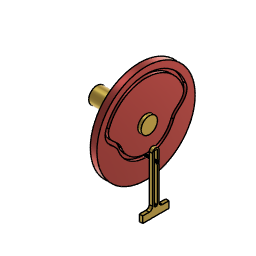
Groove Cam & Follower v1 (Autodesk Fusion 360 design; units mm, degrees)
Autodesk Fusion 360 part; units mm, degrees
sketch "Sketch1" plane through (0, 0, 0) normal (1, 0, 0) x (0, 1, 0) in component "Cam"
  circle A0 centre (0, 0) radius 150
  circle A1 centre (0, 0) radius 25
  line L0 (0, 0) -> (140.9539, 51.303) construction
  line L1 (0, 0) -> (150, 0) construction
  line L2 (0, 0) -> (140.9539, -51.303) construction
  line L3 (0, 0) -> (150, 0) construction
  line L4 (0, 0) -> (0, 44.9375) construction
  line L5 (0, 0) -> (-140.9539, 51.303) construction
  line L6 (0, 0) -> (-140.9539, -51.303) construction
  arc A2 (-84.5723, -30.7818) -> (84.5723, -30.7818) centre (0, 0) ccw
  arc A3 (-75.1754, -27.3616) -> (75.1754, -27.3616) centre (0, 0) ccw
  arc A4 (-79.8739, -29.0717) -> (79.8739, -29.0717) centre (0, 0) ccw construction
  arc A5 (112.7631, 41.0424) -> (-112.7631, 41.0424) centre (0, 0) ccw
  arc A6 (117.4616, 42.7525) -> (-117.4616, 42.7525) centre (0, 0) ccw construction
  arc A7 (122.16, 44.4626) -> (-122.16, 44.4626) centre (0, 0) ccw
  circle A8 centre (0, 0) radius 105 construction
  spline S0 degree 5 poles (79.8739, -29.0717) (80.4472, -27.4965) (81.7231, -24.4709) (84.0245, -20.3068) (87.8255, -15.4257) (93.5361, -10.0122) (99.8269, -4.7519) (106.2212, 0.8826) (112.1495, 7.2873) (116.9595, 14.6336) (119.9758, 22.9706) (120.4495, 30.4174) (119.4921, 36.4235) (118.2406, 40.6121) (117.4616, 42.7525) knots 0 0 0 0 0 0 0.1 0.2 0.3 0.4 0.5 0.6 0.7 0.8 0.9 1 1 1 1 1 1
  line L7 (76.7297, -37.7103) -> (83.0181, -20.4331)
  line L8 (121.1912, 32.5055) -> (113.732, 52.9996)
  spline S1 degree 3 poles (75.1754, -27.3616) (76.823, -22.8348) (79.1122, -18.7939) (81.8342, -15.2645) (86.0599, -9.7852) (91.2337, -5.5228) (96.2009, -1.2084) (100.1964, 2.262) (104.0844, 5.8134) (107.2713, 9.7654) (110.6099, 13.9054) (113.1413, 18.4168) (114.2898, 23.367) (115.4903, 28.5416) (115.2334, 34.2554) (112.7631, 41.0424) knots 0 0 0 0 0.154395 0.154395 0.154395 0.394087 0.394087 0.394087 0.586886 0.586886 0.586886 0.788862 0.788862 0.788862 1 1 1 1
  spline S2 degree 3 poles (84.5723, -30.7818) (86.6822, -24.985) (89.9, -20.6359) (94.2784, -16.3408) (97.8857, -12.8021) (102.2844, -9.3109) (106.7575, -5.2037) (111.1537, -1.1672) (115.5974, 3.4844) (119.026, 9.0954) (121.919, 13.8298) (124.0666, 19.2656) (124.7475, 25.2663) (125.3462, 30.5417) (124.7871, 36.2094) (122.9756, 42.0453) (122.7266, 42.8476) (122.4546, 43.6534) (122.16, 44.4626) knots 0 0 0 0 0.25 0.25 0.25 0.455973 0.455973 0.455973 0.6584 0.6584 0.6584 0.8292 0.8292 0.8292 0.979357 0.979357 0.979357 1 1 1 1
  spline S3 degree 3 poles (-75.1754, -27.3616) (-76.823, -22.8348) (-79.1122, -18.7939) (-81.8342, -15.2645) (-86.0599, -9.7852) (-91.2337, -5.5228) (-96.2009, -1.2084) (-100.1964, 2.262) (-104.0844, 5.8134) (-107.2713, 9.7654) (-110.6099, 13.9054) (-113.1413, 18.4168) (-114.2898, 23.367) (-115.4903, 28.5416) (-115.2334, 34.2554) (-112.7631, 41.0424) knots 0 0 0 0 0.154395 0.154395 0.154395 0.394087 0.394087 0.394087 0.586886 0.586886 0.586886 0.788862 0.788862 0.788862 1 1 1 1
  spline S4 degree 3 poles (-84.5723, -30.7818) (-86.6822, -24.985) (-89.9, -20.6359) (-94.2784, -16.3408) (-97.8857, -12.8021) (-102.2844, -9.3109) (-106.7575, -5.2037) (-111.1537, -1.1672) (-115.5974, 3.4844) (-119.026, 9.0954) (-121.919, 13.8298) (-124.0666, 19.2656) (-124.7475, 25.2663) (-125.3462, 30.5417) (-124.7871, 36.2094) (-122.9756, 42.0453) (-122.7266, 42.8476) (-122.4546, 43.6534) (-122.16, 44.4626) knots 0 0 0 0 0.25 0.25 0.25 0.455973 0.455973 0.455973 0.6584 0.6584 0.6584 0.8292 0.8292 0.8292 0.979357 0.979357 0.979357 1 1 1 1
  point P0 (105, 0)
  dimension "d1" = 300
  dimension "d4" = 160
  dimension "d5" = 180
  dimension "d6" = 50
  dimension "d8" = 170
  dimension "d9" = 20
  dimension "d10" = 20
  dimension "d11" = 150
  dimension "d12" = 210
  dimension "d13" = -5
  dimension "d14" = 5
  constraint coincident A0.centre A1.centre
  constraint concentric A1 A3
  constraint horizontal L1
  constraint horizontal L3
  constraint perpendicular L3 L4
  constraint symmetric A0.centre L4 A1.centre
  constraint symmetric L0.end L4 L5.end
  constraint symmetric L2.end L4 L6.end
  constraint coincident L6 A3.start
  constraint coincident L6 A2.start
  constraint coincident L5 A5.end
  constraint coincident L5 A6.end
  constraint coincident L5 A7.end
  constraint coincident L6 A4.start
  constraint coincident L0 A5.start
  constraint coincident L0 A6.start
  constraint coincident L0 A7.start
  constraint coincident L2 A2.end
  constraint coincident L2 A4.end
  constraint coincident L2 A3.end
  constraint concentric A1 A8
  constraint coincident A8 P0
  constraint coincident L1 P0
  constraint midpoint A4.end L7
  constraint tangent A4 L7
  constraint midpoint A6.start L8
  constraint tangent A6 L8
  constraint symmetric L4 A3.end A3.start
  constraint symmetric L4 A5.start A5.end
  constraint symmetric L4 S1 S3
  constraint symmetric L4 A2.end A2.start
  constraint symmetric L4 A7.start A7.end
  constraint symmetric L4 S2 S4
  measures "d1" diameter of A0
  measures "d4" diameter of A3
  measures "d5" diameter of A2
  measures "d6" diameter of A1
  measures "d8" diameter of A4
  measures "d9" angle of L0 L1
  measures "d10" angle of L2 L3
  measures "d11" distance of A0.centre L2.end
  measures "d12" diameter of A8
extrude "Extrude1" add sketch "Sketch1" along normal blind 20 makes body 1 at (0, -77.0806, 24.22) makes body 2 at (0, -121.0179, -46.6925) in component "Cam"
extrude "Extrude2" add sketch "Sketch1" along normal blind 10 contours A2 A7 S2 S4 bodies 1 2 in component "Cam"
cylinder "CylinderPrimitive1" add diameter 50 height -150 placed x (0, 0, -1) y (0, 1, 0) z (1, 0, 0) at (20, 0, 0) separate body makes body 3 in component "Axis"
move_face "OffsetFaces1" offset 10 1 faces at (20, -1.242, 6.7759) on bodies 3 in component "Axis"
ref_plane "WorkPlane1" through (50, 0, 20) normal (1, 0, 0) x (0, 1, 0) in component "Follower Base"
sketch "Sketch1 (2)" plane through (50, 0, 0) normal (1, 0, 0) x (0, 1, 0) in component "Follower Base"
  line L0 (10, -60) -> (10, -200)
  line L1 (-10, -200) -> (-10, -60)
  circle A0 centre (0, 0) radius 25
  line L2 (40, -210) -> (40, -230)
  line L3 (40, -230) -> (-40, -230)
  line L4 (-40, -230) -> (-40, -210)
  line L5 (4.8, -57.2) -> (4.8, -202.8)
  line L6 (2.8, -204.8) -> (-2.8, -204.8)
  line L7 (-4.8, -202.8) -> (-4.8, -57.2)
  line L8 (-2.8, -55.2) -> (2.8, -55.2)
  line L9 (-40, -210) -> (-20, -210)
  line L10 (20, -210) -> (40, -210)
  arc A1 (0, -50) -> (-10, -60) centre (0, -60) ccw
  arc A2 (10, -60) -> (0, -50) centre (0, -60) ccw
  arc A3 (-2.8, -55.2) -> (-4.8, -57.2) centre (-2.8, -57.2) ccw
  arc A4 (4.8, -57.2) -> (2.8, -55.2) centre (2.8, -57.2) ccw
  arc A5 (-4.8, -202.8) -> (-2.8, -204.8) centre (-2.8, -202.8) ccw
  arc A6 (2.8, -204.8) -> (4.8, -202.8) centre (2.8, -202.8) ccw
  arc A7 (-20, -210) -> (-10, -200) centre (-20, -200) ccw
  arc A8 (10, -200) -> (20, -210) centre (20, -200) ccw
  point P0 (-10, -50)
  point P1 (10, -50)
  point P2 (-10, -210)
  dimension "d23" = 20
  dimension "d24" = 160
  dimension "d25" = 10
  dimension "d27" = 80
  dimension "d28" = 20
  dimension "d29" = 30
  dimension "d31" = 10
  dimension "d32" = 2
  dimension "d33" = 2
  dimension "d34" = 10
  constraint vertical L0
  constraint vertical L1
  constraint horizontal L9
  constraint vertical L2
  constraint horizontal L3
  constraint vertical L4
  constraint collinear L9 L10
  constraint coincident P0 L1
  constraint tangent L1 A1
  constraint coincident P1 L0
  constraint tangent L0 A2
  constraint equal A1 A2
  constraint coincident A1.start A2.end
  constraint tangent L7 A3
  constraint tangent L8 A3
  constraint tangent L5 A4
  constraint tangent L8 A4
  constraint equal A3 A4
  constraint tangent L6 A5
  constraint tangent L7 A5
  constraint tangent L5 A6
  constraint tangent L6 A6
  constraint equal A5 A6
  constraint coincident P2 L1
  constraint coincident P2 L9
  constraint tangent L1 A7
  constraint tangent L9 A7
  constraint tangent L0 A8
  constraint tangent L10 A8
  constraint equal A7 A8
  measures "d23" distance of P0 P1
  measures "d24" distance of P0 P2
  measures "d25" horizontal distance of P1 A0.centre
  measures "d27" distance of L4.end L2.start
  measures "d28" distance of L4.end L3.end
  measures "d29" distance of L0 L2
  measures "d31" radius of A1
  measures "d32" radius of A3
  measures "d33" radius of A5
  measures "d34" radius of A7
extrude "Extrude1'" add sketch "Sketch1 (2)" against normal blind 10 separate body contours L0 L1 L2 L3 L4 L9 L10 A1 A2 A7 A8 makes body 4 in component "Follower Base"
sketch "Sketch1 (3)" plane through (50, 0, 0) normal (1, 0, 0) x (0, 1, 0) in component "Follower"
  arc A0 (-4.8, -202.8) -> (-2.8, -204.8) centre (-2.8, -202.8) ccw
  line L0 (-4.8, -202.8) -> (-4.8, -57.2)
  arc A1 (-2.8, -55.2) -> (-4.8, -57.2) centre (-2.8, -57.2) ccw
  line L1 (-2.8, -55.2) -> (2.8, -55.2)
  arc A2 (4.8, -57.2) -> (2.8, -55.2) centre (2.8, -57.2) ccw
  line L2 (4.8, -57.2) -> (4.8, -202.8)
  arc A3 (2.8, -204.8) -> (4.8, -202.8) centre (2.8, -202.8) ccw
  line L3 (2.8, -204.8) -> (-2.8, -204.8)
  arc A4 (10, -60) -> (-10, -60) centre (0, -60) ccw
  line L4 (-10, -60) -> (-10, -200)
  arc A5 (-20, -210) -> (-10, -200) centre (-20, -200) ccw
  line L5 (-20, -210) -> (-40, -210)
  line L6 (-40, -210) -> (-40, -230)
  line L7 (-40, -230) -> (40, -230)
  line L8 (40, -230) -> (40, -210)
  line L9 (40, -210) -> (20, -210)
  arc A6 (10, -200) -> (20, -210) centre (20, -200) ccw
  line L10 (10, -200) -> (10, -60)
  arc A7 (-75.1754, -27.3616) -> (75.1754, -27.3616) centre (0, 0) ccw
  line L11 (-4.8, -202.8) -> (-4.8, -57.2)
  line L12 (4.8, -57.2) -> (4.8, -202.8)
  circle A8 centre (0, -84.8) radius 4.8
  dimension "d37" = 9.6
  constraint tangent L0 A8
  constraint tangent A7 A8
  measures "d37" diameter of A8
extrude "Extrude1''" add sketch "Sketch1 (3)" along normal blind 10 and the other way blind 40 separate body contours A8 makes body 5 in component "Follower"
fillet "Fillet1" radius 4.5 1 edges at (60, -4.4752, -86.5358) on bodies 5 in component "Follower"
component "Follower" placed x (1, 0, 0) y (0, 1, 0) z (0, 0, 1) at (0, 0, 0)
component "Cam" placed x (1, 0, 0) y (0, 1, 0) z (0, 0, 1) at (0, 0, 0)
component "Axis" placed x (1, 0, 0) y (0, 1, 0) z (0, 0, 1) at (0, 0, 0)
component "Follower Base" placed x (1, 0, 0) y (0, 1, 0) z (0, 0, 1) at (0, 0, 0)
